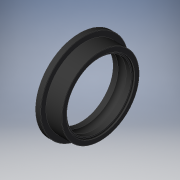
# Autodesk Inventor part: SKF_W 61900 R-2RS1_PART2
Saved by Autodesk Inventor 2019 (Build 230136000, 136)
## iProperties
Created: 2022-08-03
Part Number: SKF_W 61900 R-2RS1_PART2
Material: Generic
Catalog Web Link: www.cadenas.de
Description: -Deep groove ball bearings
Vendor: SKF
Document SubType Name: Modeling
Designer: psAdmin
Manufacturer: SKF
Mass: 11 g
Surface Area: 12.3168 cm^2
Volume: 0.810933 cm^3
Density: 1 g/cm^3
Appearance: PSOLRGB-175-175-175
Category: PARTsolutions
Company: SKF
Title: SKF_W 61900 R-2RS1_PART2
Author: Cadenas PARTsolutions
Comments: Deep groove ball bearings
PSOL_IDENT_0: {$CADENAS_DATA/23d-libs/skf/bearings_units_and_housings/ball_bearings/deep_groove_ball_bearings/bb1_
PSOL_IDENT_1: 001_101.prj},215 {VTYP=3D},{NB=SKF_W 61900 R-2RS1_PART2},{LINA=SKF_W 61900 R-2RS1_PART2},{NN=BB1_001
PSOL_IDENT_2: _101_PART2},{NOPRJ=TRUE},{DATE=29.07.2022 12:16:16},{GEOMDATE=04.07.2022 10:54:51},{VERSION=},{LINEI
PSOL_IDENT_3: D=21610},{WBVAR=},{WBNUMERIC=}  {NB=SKF_W 61900 R-2RS1_PART2},{LINA=SKF_W 61900 R-2RS1_PART2},{KT=DU
PSOL_IDENT_4: MMY},{DESIGNATION=W 61900 R-2RS1},{R12=0.30},{DD=10.000},{D=22.000},{B=6.000},{C=},{CX=},{CXX=1.5},{
PSOL_IDENT_5: CA=1.500},{XXVARIANT=Flanged outer ring},{XXDESIGN=Single row stainless steel},{XXSEALING=Contact se
PSOL_IDENT_6: al on both sides},{DESIGN=dgbbwr2zs},{DESIGNIR=dgbbwr2zs},{VARIANT=Flanged outer ring},{DD1=13.90},{
PSOL_IDENT_7: DD2=13.2},{DD2X=},{DD2A=13.20},{D1=18.20},{D1X=0.00},{D2=19.4},{D2A=19.40},{D3=25},{D3X=},{D3A=25.00
PSOL_IDENT_8: 0},{D4=},{HH=0.000},{BB=0.000},{BBX=},{BBA=0.000},{FF=},{R0MAX=0.000},{R0=0.000},{PITCH=16.00},{DW=3
PSOL_IDENT_9: .175},{DDAMIN=12.000},{DDAMAX=13.000},{DDBMIN=0.000},{DDBMAX=0.000},{DBMIN=0.000},{DAMAX=0.000},{BBA
PSOL_IDENT_10: MIN=0.000},{CAMAX=0.000},{RAMAX=0.300},{LOAD1=2.340},{LOAD2=1.250},{LOAD3=0.054},{SPEED1=0},{SPEED2=
PSOL_IDENT_11: 20000},{KR=0.025},{F0=14.000},{Z=9},{II=1},{MASS=0.011},{BEARING=W 61900 R-2RS1},{RING=},{HELP=1.900
PSOL_IDENT_12: },{HELP2=1.300},{DD1ALG=6.950},{YALG=6.950},{PITCH1=16.000},{DW1=3.175},{YALG1=9.100},{HALG1=1.900},
PSOL_IDENT_13: {SH=6.600},{CU=0.565},{HALG=1.95},{B1=-3.22875},{SHIELDHELP=2},{D4A=0.000},{FFA=0.000},{RS1=},{HELP3=
PSOL_IDENT_14: 0}
NB: SKF_W 61900 R-2RS1_PART2
NT: Deep groove ball bearings
NBSYN: SKF_$DESIGNATION._PART2
LINA: SKF_W 61900 R-2RS1_PART2
CATALOG: SKF
DESIGNATION: W 61900 R-2RS1
R12: 0.3
DD: 10
D: 22
B: 6
XXVARIANT: Flanged outer ring
XXDESIGN: Single row stainless steel
XXSEALING: Contact seal on both sides
DD2: 13.2
D2: 19.4
LOAD1: 2.34
LOAD2: 1.25
LOAD3: 0.054
SPEED1: 0
SPEED2: 20000
BEARING: W 61900 R-2RS1
SUPPLIER: SKF
ARTICLENO: SKF_W 61900 R-2RS1_PART2
BOMINFO: SKF_W 61900 R-2RS1_PART2
CREATOR: CADENAS GmbH
Autodesk Inventor part; units mm, degrees
ref_plane "YZ Plane" through (0, 0, 0) normal (1, 0, 0) x (0, 1, 0)
ref_plane "XZ Plane" through (0, 0, 0) normal (0, 1, 0) x (-1, 0, 0)
ref_plane "XY Plane" through (0, 0, 0) normal (0, 0, 1) x (1, 0, 0)
sketch "Sketch_21" plane through (0, 0, 0) normal (0, 0, 1) x (1, 0, 0)
  line L0 (50, 0) -> (-50, 0)
  line L1 (0, 12.4) -> (0, 9.7)
  line L2 (0, 9.7) -> (0.15, 9.7)
  arc A0 (0.45, 9.4) -> (0.15, 9.7) centre (0.15, 9.4) ccw
  line L3 (0.45, 9.4) -> (0.45, 9.1)
  line L4 (0.45, 9.1) -> (1.8554, 9.1)
  arc A1 (4.1446, 9.1) -> (1.8554, 9.1) centre (3, 8) ccw
  line L5 (4.1446, 9.1) -> (5.55, 9.1)
  line L6 (5.55, 9.1) -> (5.55, 9.4)
  arc A2 (5.85, 9.7) -> (5.55, 9.4) centre (5.85, 9.4) ccw
  line L7 (5.85, 9.7) -> (6, 9.7)
  line L8 (6, 9.7) -> (6, 10.9)
  arc A3 (6, 10.9) -> (5.9, 11) centre (5.9, 10.9) ccw
  line L9 (5.9, 11) -> (1.5, 11)
  line L10 (1.5, 11) -> (1.5, 12.4)
  arc A4 (1.5, 12.4) -> (1.4, 12.5) centre (1.4, 12.4) ccw
  line L11 (1.4, 12.5) -> (0.1, 12.5)
  arc A5 (0.1, 12.5) -> (0, 12.4) centre (0.1, 12.4) ccw
  constraints: 24 end point, 12 point on circle, 6 centre point
revolve "Revolution1" add sketch "Sketch_21" angle 360 about axis through (50, 0, 0) along (1, 0, 0)
body "Solid1"
